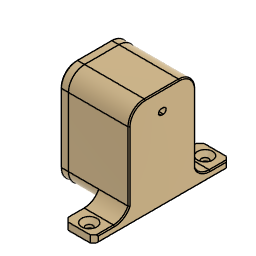
Suporte boia 2 v8 (Autodesk Fusion 360 design; units mm, degrees)
Autodesk Fusion 360 part; units mm, degrees
sketch "Sketch1" plane through (0, 0, 0) normal (1, 0, 0) x (0, 1, 0)
  line L0 (8, 0) -> (25, 0)
  line L1 (33, 8) -> (33, 42)
  arc A0 (33, 42) -> (25, 50) centre (25, 42) ccw
  line L2 (25, 50) -> (8, 50)
  arc A1 (8, 50) -> (0, 42) centre (8, 42) ccw
  line L3 (0, 42) -> (0, 8)
  line L4 (16.5, 50) -> (16.5, 30) construction
  circle A2 centre (16.5, 30) radius 6.25
  arc A3 (0, 8) -> (8, 0) centre (8, 8) ccw
  arc A4 (25, 0) -> (33, 8) centre (25, 8) ccw
  line L5 (8, 2.5) -> (25, 2.5)
  arc A5 (25, 2.5) -> (30.5, 8) centre (25, 8) ccw
  line L6 (30.5, 8) -> (30.5, 42)
  arc A6 (30.5, 42) -> (25, 47.5) centre (25, 42) ccw
  line L7 (25, 47.5) -> (8, 47.5)
  arc A7 (8, 47.5) -> (2.5, 42) centre (8, 42) ccw
  line L8 (2.5, 42) -> (2.5, 8)
  arc A8 (2.5, 8) -> (8, 2.5) centre (8, 8) ccw
  line L9 (8, 5) -> (25, 5)
  arc A9 (25, 5) -> (28, 8) centre (25, 8) ccw
  line L10 (28, 8) -> (28, 42)
  arc A10 (28, 42) -> (25, 45) centre (25, 42) ccw
  line L11 (25, 45) -> (8, 45)
  arc A11 (8, 45) -> (5, 42) centre (8, 42) ccw
  line L12 (5, 42) -> (5, 8)
  arc A12 (5, 8) -> (8, 5) centre (8, 8) ccw
  point P0 (33, 0)
  dimension "d1" = 8
  dimension "d2" = 12.5
  dimension "d3" = 30
  dimension "d4" = 50
  dimension "d5" = 33
  dimension "d34" = 8
  dimension "d35" = -2.5
  dimension "d36" = -5
  constraint horizontal L0
  constraint perpendicular L0 L1
  constraint tangent L1 A0
  constraint parallel L0 L2
  constraint tangent L2 A1
  constraint equal A0 A1
  constraint tangent A1 L3
  constraint tangent A0 L2
  constraint vertical L3
  constraint midpoint L2 L4.start
  constraint perpendicular L2 L4
  constraint coincident L4.end A2.centre
  constraint coincident origin L0
  constraint coincident origin L3
  constraint tangent L0 A3
  constraint tangent L3 A3
  constraint coincident P0 L0
  constraint coincident P0 L1
  constraint tangent L0 A4
  constraint tangent L1 A4
  constraint equal A3 A4
  measures "d1" radius of A0
  measures "d2" diameter of A2
  measures "d3" distance of L0 L4.end
  measures "d4" distance of L0 L2
  measures "d5" distance of origin P0
  measures "d34" radius of A3
extrude "Extrude1" add sketch "Sketch1" against normal blind 4 contours L0 L1 A0 L2 A1 L3 A3 A4 | L5 A5 L6 A6 L7 A7 L8 A8 | L9 A9 L10 A10 L11 A11 L12 A12 makes body 1
extrude "Extrude3" add sketch "Sketch1" along normal blind 2 contours L5 A5 L6 A6 L7 A7 L8 A8 bodies 1
extrude "Extrude8" add sketch "Sketch1" along normal blind 30 separate body contours L0 L1 A0 L2 A1 L3 A3 A4 | A2 | L5 A5 L6 A6 L7 A7 L8 A8 | L9 A9 L10 A10 L11 A11 L12 A12 makes body 2
combine "Combine2" operation cut target body 2 tool bodies 1 keep tools
extrude "Extrude9" cut sketch "Sketch1" along normal up to surface (26 mm away) contours A2 | L9 A9 L10 A10 L11 A11 L12 A12 bodies 2
extrude "Extrude10" cut 1 faces at (2, 4.1667, 30.6667) along direction (1, 0, 0) up to surface (20 mm away) from surface at 4 on bodies 2 bodies 2
chamfer "Chamfer2" distance 2.5 angle 45 8 edges at (6, 28.8891, 45.8891) (6, 16.5, 47.5) (6, 4.1109, 45.8891) (6, 2.5, 25) (6, 4.1109, 4.1109) (6, 16.5, 2.5) (6, 28.8891, 4.1109) (6, 30.5, 25) on bodies 2
sketch "Sketch4" plane through (30, 0, 0) normal (1, 0, 0) x (0, 1, 0)
  arc A0 (25, 0) -> (33, 8) centre (25, 8) ccw
  line L0 (33, 8) -> (33, 42)
  arc A1 (33, 42) -> (25, 50) centre (25, 42) ccw
  line L1 (25, 50) -> (8, 50)
  arc A2 (8, 50) -> (0, 42) centre (8, 42) ccw
  line L2 (0, 42) -> (0, 8)
  arc A3 (0, 8) -> (8, 0) centre (8, 8) ccw
  line L3 (8, 0) -> (25, 0)
  line L4 (16, 39.2) -> (17, 39.2)
  arc A4 (17, 39.2) -> (17, 42) centre (17, 40.6) ccw
  line L5 (17, 42) -> (16, 42)
  arc A5 (16, 42) -> (16, 39.2) centre (16, 40.6) ccw
  line L6 (16, 40.6) -> (17, 40.6) construction
  line L7 (16.5, 42) -> (16.5, 50) construction
  dimension "d45" = 8
  dimension "d46" = 1.4
  dimension "d47" = 1
  constraint tangent L4 A4
  constraint tangent A4 L5
  constraint parallel L4 L5
  constraint tangent L5 A5
  constraint tangent L4 A5
  constraint parallel L1 L6
  constraint midpoint L5 L7.start
  constraint midpoint L1 L7.end
  constraint vertical L7
  measures "d45" distance of L7.start L7.end
  measures "d46" radius of A4
  measures "d47" distance of L4.start L4.end
extrude "Extrude11" cut sketch "Sketch4" against normal blind 5 contours L4 A4 L5 A5 bodies 2
sketch "Esboço5" plane through (30, 0, 0) normal (1, 0, 0) x (0, 1, 0)
  line L0 (17, 39.2) -> (16, 39.2)
  arc A0 (16, 42) -> (16, 39.2) centre (16, 40.6) ccw
  line L1 (16, 42) -> (17, 42)
  arc A1 (17, 39.2) -> (17, 42) centre (17, 40.6) ccw
  arc A2 (25, 0) -> (33, 8) centre (25, 8) ccw
  line L2 (33, 8) -> (33, 42)
  arc A3 (33, 42) -> (25, 50) centre (25, 42) ccw
  line L3 (25, 50) -> (8, 50)
  arc A4 (8, 50) -> (0, 42) centre (8, 42) ccw
  line L4 (0, 42) -> (0, 8)
  arc A5 (0, 8) -> (8, 0) centre (8, 8) ccw
  line L5 (8, 0) -> (25, 0)
  line L6 (8, 0) -> (-17.1937, 0)
  line L7 (-17.1937, 0) -> (-17.1937, 3.5)
  line L8 (-17.1937, 3.5) -> (-7.1937, 3.5)
  arc A6 (-7.1937, 3.5) -> (0, 8) centre (-7.1937, 11.5) ccw
  line L9 (16.5, 0) -> (16.5, -9.2763) construction
  arc A7 (33, 8) -> (40.1937, 3.5) centre (40.1937, 11.5) ccw
  line L10 (50.1937, 3.5) -> (40.1937, 3.5)
  line L11 (50.1937, 0) -> (50.1937, 3.5)
  line L12 (25, 0) -> (50.1937, 0)
  dimension "d50" = 3.5
  dimension "d51" = 10
  dimension "d52" = 8
  constraint coincident A5.end L5.start
  constraint tangent A5 L6
  constraint perpendicular L6 L7
  constraint perpendicular L7 L8
  constraint coincident L4 A5.start
  constraint tangent L8 A6
  constraint coincident L4.end A5.start
  constraint midpoint L5 L9.start
  constraint perpendicular L5 L9
  constraint symmetric A5.end L9 A2.start
  constraint symmetric L6.end L9 L11.start
  constraint symmetric L7.end L9 L10.start
  constraint symmetric L8.end L9 A7.end
  constraint symmetric L4.end L9 A2.end
  constraint symmetric A6 L9 A7
  measures "d50" distance of L6.end L7.end
  measures "d51" distance of L7.end L8.end
  measures "d52" radius of A6
extrude "Extrusão12" add sketch "Esboço5" against normal blind 15 contours A2 A7 L10 L11 L12 | A5 L6 L7 L8 A6 bodies 2
sketch "Esboço6" plane through (0, 0, 3.5) normal (0, 0, 1) x (-1, 0, 0)
  line L0 (-30, 17.1937) -> (-30, 7.1937)
  line L1 (-30, 7.1937) -> (-15, 7.1937)
  line L2 (-15, 7.1937) -> (-15, 17.1937)
  line L3 (-15, 17.1937) -> (-30, 17.1937)
  line L4 (-30, 17.1937) -> (-15, 7.1937) construction
  line L5 (-30, -40.1937) -> (-30, -50.1937)
  line L6 (-30, -50.1937) -> (-15, -50.1937)
  line L7 (-15, -50.1937) -> (-15, -40.1937)
  line L8 (-15, -40.1937) -> (-30, -40.1937)
  line L9 (-15, -50.1937) -> (-30, -40.1937) construction
  circle A0 centre (-22.5, -45.1937) radius 1.75
  circle A1 centre (-22.5, 12.1937) radius 1.75
  dimension "d55" = 3.5
  constraint coincident L0.start L3.end
  constraint coincident L1.end L2.start
  constraint coincident L6.end L7.start
  constraint coincident L5.start L8.end
  constraint midpoint L9 A0.centre
  constraint midpoint L4 A1.centre
  constraint equal A0 A1
  measures "d55" diameter of A0
extrude "Extrusão13" cut sketch "Esboço6" against normal blind 10 contours A0 | A1 bodies 2
chamfer "Chanfro3" distance 2 angle 45 2 edges at (24.1316, 44.5609, 3.5) (24.1316, -12.8266, 3.5) on bodies 2
chamfer "Chanfro4" distance 2 angle 45 4 edges at (30, -17.1937, 1.75) (15, -17.1937, 1.75) (30, 50.1937, 1.75) (15, 50.1937, 1.75) on bodies 2
chamfer "Chamfer5" distance 0.5 angle 45 18 edges at (-4, 2.3431, 47.6569) (-4, 16.5, 50) (-4, 30.6569, 47.6569) (-4, 33, 25) (-4, 30.6569, 2.3431) (-4, 16.5, 0) (-4, 2.3431, 2.3431) (-4, 0, 25) (30, 2.3431, 47.6569) (30, 0, 25) (30, 33, 25) (30, 30.6569, 47.6569) (30, 16.5, 50) (30, 16.5, 0) (30, -2.9511, 4.7177) (30, -11.1937, 3.5) (30, 35.9511, 4.7177) (30, 44.1937, 3.5) on bodies 1 2
